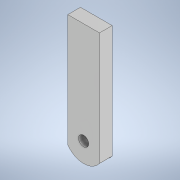
# Autodesk Inventor part: Throttle Arm
Saved by Autodesk Inventor 2020.4 (Build 244396000, 396)
## iProperties
Created: 2022-04-15
Part Number: Throttle Arm
Material: Aluminum 6061-AHC
Document SubType Name: Modeling
Designer: Gurkin
Density: 2.7 g/cm^3
Appearance: Aluminum - Dark
Author: Gurkin
Autodesk Inventor part; units mm, degrees
ref_plane "YZ Plane" through (0, 0, 0) normal (1, 0, 0) x (0, 1, 0)
ref_plane "XZ Plane" through (0, 0, 0) normal (0, 1, 0) x (-1, 0, 0)
ref_plane "XY Plane" through (0, 0, 0) normal (0, 0, 1) x (1, 0, 0)
sketch "Sketch1" plane through (0, 0, 0) normal (0, 0, 1) x (1, 0, 0)
  line L0 (-25, 160) -> (25, 160)
  line L1 (25, 160) -> (25, -18)
  line L2 (-25, 160) -> (-25, -18)
  arc A0 (-25, -18) -> (25, -18) centre (0, 0) ccw
  dimension "d62" = 90
  dimension "d63" = 160
  dimension "d64" = 50
  dimension "d65" = 18
  constraints: 6 end point, 2 parallel, 2 point on circle, 1 centre point, 1 coincident, 1 horizontal
  measures "d62" angle of L1 L0
  measures "d63" distance from line of point (0, 0) L0
  measures "d64" distance between parallel lines of L2 L1
  measures "d65" vertical distance of L2.end point (0, 0)
extrude "Extrusion1" add sketch "Sketch1" along normal blind 20
sketch "Sketch10" plane through (0, 0, 0) normal (0, 0, -1) x (-1, 0, 0)
  circle A0 centre (0, 0) radius 8
  dimension "d54" = 16
  constraints: 1 centre point, 1 coincident
  measures "d54" diameter of A0
extrude "Extrusion7" cut sketch "Sketch10" against normal through all
body "Solid1"
